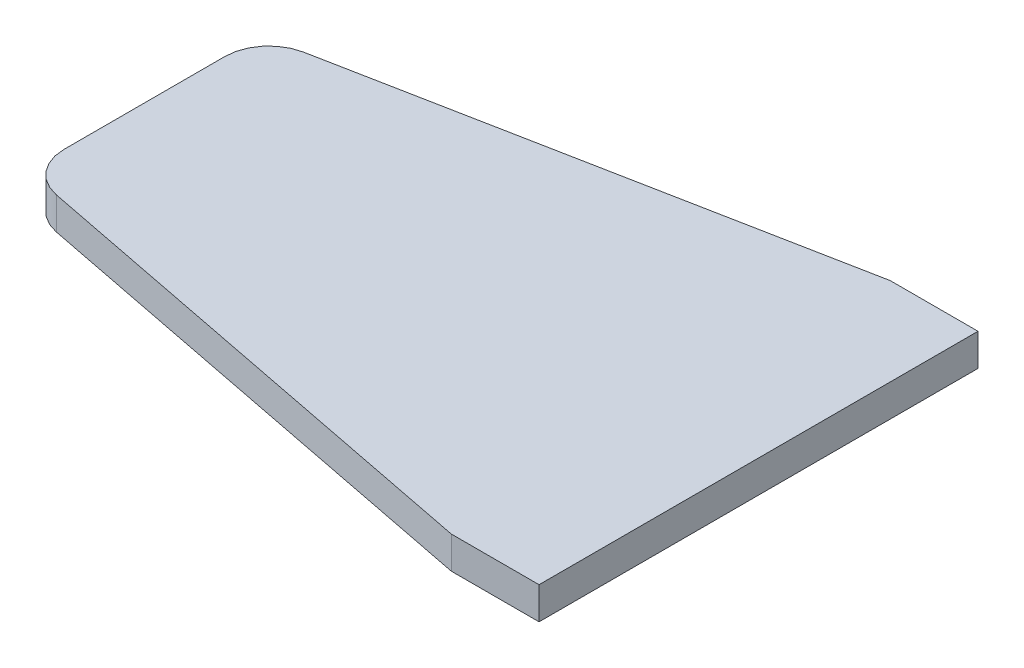
# Autodesk Inventor part: porte-girouette
Saved by Autodesk Inventor 2020 (Build 240168000, 168)
## iProperties
Created: 2019-10-24
Part Number: porte-girouette
Material: Générique
Document SubType Name: Modeling
Designer: erwan
Density: 1 g/cm^3
Appearance: Par défaut
Author: erwan
Autodesk Inventor part; units mm, degrees
ref_plane "YZ Plane" through (0, 0, 0) normal (1, 0, 0) x (0, 1, 0)
ref_plane "XZ Plane" through (0, 0, 0) normal (0, 1, 0) x (-1, 0, 0)
ref_plane "XY Plane" through (0, 0, 0) normal (0, 0, 1) x (1, 0, 0)
sketch "Esquisse1" plane through (0, 0, 0) normal (0, 1, 0) x (-1, 0, 0)
  line L0 (0, 0) -> (60, 0)
  line L1 (60, -300) -> (0, -300)
  line L2 (0, -300) -> (0, 0)
  line L3 (60, 0) -> (129.2506, -13.461) construction
  line L4 (60, -300) -> (124.1651, -287.5276) construction
  line L5 (60, 0) -> (420, -70.5468)
  line L6 (60, -300) -> (420, -230.0231)
  line L7 (420, -70.5468) -> (420, -230.0231)
  line L8 (60, 0) -> (60, -300) construction
  dimension "d0" = 300
  dimension "d1" = 60
  dimension "d5" = 420
  constraints: 18 end point, 2 vertical, 1 coincident, 1 horizontal, 1 parallel, 1 point on line
  measures "d0" distance of L0.end L1.start
  measures "d1" distance of L0.start L0.end
  measures "d5" distance from line of L2 L6.end
extrude "Extrusion1" add sketch "Esquisse1" along normal blind 22
fillet "Congé1" radius 30 2 edges at (-420, 11, -70.5468) (-420, 11, -230.0231)
